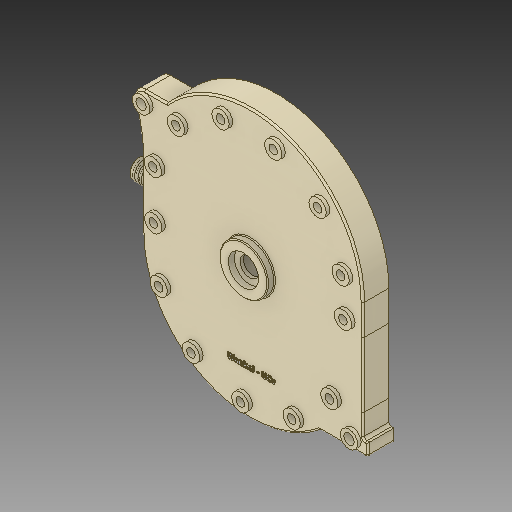
# Autodesk Inventor part: CapacFata
Saved by Autodesk Inventor 2019.4 (Build 234330000, 330)
## iProperties
Created: 2020-05-01
Part Number: CapacFata
Material: Aluminum 6061-AHC
Document SubType Name: Modeling
Designer: Gabriel
Density: 2.7 g/cm^3
Appearance: Light Beige
Author: Gabriel
Autodesk Inventor part; units mm, degrees
sketch "Sketch1" plane through (0, 0, 0) normal (0, 0, 1) x (1, 0, 0)
  arc A0 (-129.637, -28.0388) -> (75.3644, -124.0845) centre (-4.637, -28.0388) ccw projected
  line L0 (128.3644, -124.0845) -> (75.3644, -124.0845) projected
  line L1 (-129.637, -28.0388) -> (-129.637, 41.9612) projected
  arc A1 (-129.637, 41.9612) -> (-138.5073, 99.3374) centre (-319.637, 41.9612) ccw projected
  arc A2 (-127.0676, 114.9612) -> (-138.5073, 99.3374) centre (-127.0676, 102.9612) ccw projected
  line L2 (-127.0676, 114.9612) -> (-101.2341, 114.9612) projected
  arc A3 (125.363, 27.9662) -> (-101.2341, 114.9612) centre (-4.637, 27.9612) ccw projected
  line L3 (125.363, 27.9662) -> (125.3643, -7.0846) projected
  line L4 (125.3644, -106.0845) -> (125.3644, -82.0845) projected
  arc A4 (125.3644, -106.0845) -> (128.3644, -109.0845) centre (128.3644, -106.0845) ccw projected
  line L5 (131.3644, -109.0845) -> (131.3644, -121.0845) projected
  line L6 (131.3644, -109.0845) -> (128.3644, -109.0845) projected
  arc A5 (128.3644, -124.0845) -> (131.3644, -121.0845) centre (128.3644, -121.0845) ccw projected
  circle A6 centre (113.3644, -112.0845) radius 6 projected
  circle A7 centre (-127.0676, 102.9612) radius 6 projected
  line L7 (125.3643, -7.0846) -> (125.3644, -82.0845)
  constraints: 2 end point
extrude "Extrusion1" add sketch "Sketch1" along normal blind 30
ref_plane "Work Plane1" through (0, 0, 14) normal (0, 0, 1) x (1, 0, 0)
sketch "Sketch2" plane through (0, 0, 14) normal (0, 0, 1) x (1, 0, 0)
  circle A0 centre (-86.7234, 101.7852) radius 5 projected
  circle A1 centre (-35.1294, 134.0667) radius 5 projected
  circle A2 centre (25.7313, 134.1022) radius 5 projected
  circle A3 centre (77.1089, 101.5656) radius 5 projected
  circle A4 centre (103.6918, 47.0625) radius 5 projected
  circle A5 centre (106.363, 3.9612) radius 5 projected
  circle A6 centre (90.6258, -83.0388) radius 5 projected
  circle A7 centre (47.0048, -125.1631) radius 5 projected
  circle A8 centre (-12.3102, -137.7709) radius 5 projected
  circle A9 centre (-69.2934, -117.0307) radius 5 projected
  circle A10 centre (-106.6272, -69.2455) radius 5 projected
  circle A11 centre (-112.9659, -8.9375) radius 5 projected
  circle A12 centre (-113.371, 47.0684) radius 5 projected
extrude "Extrusion2" cut sketch "Sketch2" against normal through all
sketch "Sketch3" plane through (0, 0, 14) normal (0, 0, 1) x (1, 0, 0)
  circle A0 centre (-86.7234, 101.7852) radius 5 projected
  circle A1 centre (25.7313, 134.1022) radius 5 projected
  circle A2 centre (77.1089, 101.5656) radius 5 projected
  circle A3 centre (-35.1294, 134.0667) radius 5 projected
  circle A4 centre (-113.371, 47.0684) radius 5 projected
  line L0 (96.363, 34.1163) -> (96.363, 14.2081) projected
  arc A5 (96.363, 14.2081) -> (99.5937, 12.6317) centre (98.363, 14.2081) ccw projected
  arc A6 (112.2861, 13.2303) -> (99.5937, 12.6317) centre (106.363, 3.9612) ccw projected
  arc A7 (112.2861, 13.2303) -> (115.363, 14.9156) centre (113.363, 14.9156) ccw projected
  line L1 (115.363, 14.9156) -> (115.363, 36.9398) projected
  arc A8 (115.363, 36.9398) -> (111.9814, 38.3859) centre (113.363, 36.9398) ccw projected
  arc A9 (99.1242, 35.9658) -> (111.9814, 38.3859) centre (103.6918, 47.0625) ccw projected
  arc A10 (99.1242, 35.9658) -> (96.363, 34.1163) centre (98.363, 34.1163) ccw projected
  line L2 (118.363, -28.0388) -> (118.363, 27.9612) projected
  arc A11 (-127.637, -28.0388) -> (118.363, -28.0388) centre (-4.637, -28.0388) ccw projected
  line L3 (-127.637, 27.9612) -> (-127.637, -28.0388) projected
  arc A12 (118.363, 27.9612) -> (-127.637, 27.9612) centre (-4.637, 27.9612) ccw projected
  line L4 (115.363, -10.6889) -> (115.363, -8.6879) projected
  arc A13 (115.363, -8.6879) -> (111.0773, -5.9774) centre (112.363, -8.6879) ccw projected
  arc A14 (100.863, -5.5651) -> (111.0773, -5.9774) centre (106.363, 3.9612) ccw projected
  arc A15 (100.863, -5.5651) -> (96.363, -8.1632) centre (99.363, -8.1632) ccw projected
  line L5 (96.363, -8.1632) -> (96.363, -28.0388) projected
  arc A16 (88.1817, -67.8595) -> (96.363, -28.0388) centre (-4.637, -28.0388) ccw projected
  arc A17 (88.1817, -67.8595) -> (90.8716, -72.0416) centre (90.9387, -69.0423) ccw projected
  arc A18 (99.8396, -77.03) -> (90.8716, -72.0416) centre (90.6258, -83.0388) ccw projected
  arc A19 (99.8396, -77.03) -> (105.0958, -76.6054) centre (102.3524, -75.3913) ccw projected
  arc A20 (105.0958, -76.6054) -> (115.363, -28.0388) centre (-4.637, -28.0388) ccw projected
  line L6 (115.363, -28.0388) -> (115.363, -22.0845) projected
  line L7 (109.363, -22.0845) -> (115.363, -22.0845) projected
  line L8 (109.363, -12.6889) -> (109.363, -22.0845) projected
  arc A21 (111.363, -10.6889) -> (109.363, -12.6889) centre (111.363, -12.6889) ccw projected
  line L9 (115.363, -10.6889) -> (111.363, -10.6889) projected
  line L10 (-105.637, 4.3764) -> (-105.637, 33.9465) projected
  arc A22 (-105.637, 33.9465) -> (-109.6029, 36.7868) centre (-108.637, 33.9465) ccw projected
  arc A23 (-119.8172, 38.4561) -> (-109.6029, 36.7868) centre (-113.1445, 47.2011) ccw projected
  arc A24 (-119.8172, 38.4561) -> (-124.637, 36.0711) centre (-121.637, 36.0711) ccw projected
  line L11 (-124.637, 36.0711) -> (-124.637, 2.0539) projected
  arc A25 (-124.637, 2.0539) -> (-119.7789, -0.3014) centre (-121.637, 2.0539) ccw projected
  arc A26 (-109.5646, 1.5234) -> (-119.7789, -0.3014) centre (-112.9659, -8.9375) ccw projected
  arc A27 (-109.5646, 1.5234) -> (-105.637, 4.3764) centre (-108.637, 4.3764) ccw projected
  arc A28 (-119.5689, -17.7352) -> (-108.6305, -19.0472) centre (-112.9659, -8.9375) ccw projected
  arc A29 (-119.5689, -17.7352) -> (-124.3629, -19.932) centre (-121.3697, -20.1346) ccw projected
  arc A30 (-124.3629, -19.932) -> (-120.0611, -60.8609) centre (-4.637, -28.0388) ccw projected
  arc A31 (-120.0611, -60.8609) -> (-114.9151, -62.0129) centre (-117.1755, -60.0404) ccw projected
  arc A32 (-104.4886, -58.4555) -> (-114.9151, -62.0129) centre (-106.6272, -69.2455) ccw projected
  arc A33 (-104.4886, -58.4555) -> (-101.014, -54.7125) centre (-103.9053, -55.5127) ccw projected
  arc A34 (-104.4537, -21.9859) -> (-101.014, -54.7125) centre (-4.637, -28.0388) ccw projected
  arc A35 (-104.4537, -21.9859) -> (-108.6305, -19.0472) centre (-107.4482, -21.8043) ccw projected
  arc A36 (-107.5648, -80.2055) -> (-97.5934, -75.5216) centre (-106.6272, -69.2455) ccw projected
  arc A37 (-107.5648, -80.2055) -> (-110.4663, -84.6088) centre (-107.8206, -83.1946) ccw projected
  arc A38 (-110.4663, -84.6088) -> (-85.1291, -117.039) centre (-4.637, -28.0388) ccw projected
  arc A39 (-85.1291, -117.039) -> (-80.1546, -115.289) centre (-83.1168, -114.814) ccw projected
  arc A40 (-73.1976, -106.7468) -> (-80.1546, -115.289) centre (-69.2934, -117.0307) ccw projected
  arc A41 (-73.1976, -106.7468) -> (-72.2344, -101.7314) centre (-74.2623, -103.9422) ccw projected
  arc A42 (-92.4939, -75.8004) -> (-72.2344, -101.7314) centre (-4.637, -28.0388) ccw projected
  arc A43 (-92.4939, -75.8004) -> (-97.5934, -75.5216) centre (-95.1296, -77.2333) ccw projected
  arc A44 (-64.2806, -126.8221) -> (-58.3064, -117.5659) centre (-69.2934, -117.0307) ccw projected
  arc A45 (-64.2806, -126.8221) -> (-64.4078, -132.0939) centre (-62.9135, -129.4925) ccw projected
  arc A46 (-64.4078, -132.0939) -> (-25.7353, -146.1695) centre (-4.637, -28.0388) ccw projected
  arc A47 (-25.7353, -146.1695) -> (-22.4441, -142.0494) centre (-25.2078, -143.2163) ccw projected
  arc A48 (-21.0708, -131.1186) -> (-22.4441, -142.0494) centre (-12.3102, -137.7709) ccw projected
  arc A49 (-21.0708, -131.1186) -> (-22.9118, -126.3548) centre (-23.46, -129.3043) ccw projected
  arc A50 (-53.8341, -115.1) -> (-22.9118, -126.3548) centre (-4.637, -28.0388) ccw projected
  arc A51 (-53.8341, -115.1) -> (-58.3064, -117.5659) centre (-55.31, -117.7118) ccw projected
  arc A52 (-2.8705, -143.4181) -> (-2.7091, -132.4025) centre (-12.3102, -137.7709) ccw projected
  arc A53 (-2.8705, -143.4181) -> (-0.1847, -147.9562) centre (-0.296, -144.9583) ccw projected
  arc A54 (-0.1847, -147.9562) -> (40.0704, -139.3997) centre (-4.637, -28.0388) ccw projected
  arc A55 (40.0704, -139.3997) -> (40.6782, -134.1615) centre (38.9527, -136.6157) ccw projected
  arc A56 (36.0503, -124.1639) -> (40.6782, -134.1615) centre (47.0048, -125.1631) ccw projected
  arc A57 (36.0503, -124.1639) -> (31.9647, -121.0996) centre (33.0627, -123.8915) ccw projected
  arc A58 (-0.2231, -127.9414) -> (31.9647, -121.0996) centre (-4.637, -28.0388) ccw projected
  arc A59 (-0.2231, -127.9414) -> (-2.7091, -132.4025) centre (-0.0907, -130.9384) ccw projected
  arc A60 (80.8064, -87.9965) -> (90.0289, -94.0226) centre (90.6258, -83.0388) ccw projected
  arc A61 (80.8064, -87.9965) -> (75.7177, -87.5629) centre (78.1283, -89.3487) ccw projected
  arc A62 (52.0465, -110.4219) -> (75.7177, -87.5629) centre (-4.637, -28.0388) ccw projected
  arc A63 (52.0465, -110.4219) -> (52.3022, -115.5226) centre (53.747, -112.8934) ccw projected
  arc A64 (58.0028, -124.9499) -> (52.3022, -115.5226) centre (47.0048, -125.1631) ccw projected
  arc A65 (58.0028, -124.9499) -> (62.6853, -127.3752) centre (61.0022, -124.8917) ccw projected
  arc A66 (62.6853, -127.3752) -> (92.2893, -98.7869) centre (-4.637, -28.0388) ccw projected
  arc A67 (92.2893, -98.7869) -> (90.0289, -94.0226) centre (89.8661, -97.0182) ccw projected
  arc A68 (-105.5908, 54.8446) -> (-116.2183, 57.6935) centre (-113.371, 47.0684) ccw projected
  arc A69 (-105.5908, 54.8446) -> (-100.5904, 56.1206) centre (-103.469, 56.9654) ccw projected
  arc A70 (-86.0788, 85.9891) -> (-100.5904, 56.1206) centre (-4.637, 27.9612) ccw projected
  arc A71 (-86.0788, 85.9891) -> (-88.0637, 90.6947) centre (-88.522, 87.7299) ccw projected
  arc A72 (-96.6447, 97.6037) -> (-88.0637, 90.6947) centre (-86.383, 101.5656) ccw projected
  arc A73 (-96.6447, 97.6037) -> (-101.8743, 98.2812) centre (-99.4434, 96.5232) ccw projected
  arc A74 (-101.8743, 98.2812) -> (-119.8758, 61.4279) centre (-4.637, 27.9612) ccw projected
  arc A75 (-119.8758, 61.4279) -> (-116.2183, 57.6935) centre (-116.9948, 60.5913) ccw projected
  arc A76 (-76.0047, 104.257) -> (-83.5076, 112.3047) centre (-86.7234, 101.7852) ccw projected
  arc A77 (-76.0047, 104.257) -> (-71.0879, 102.6893) centre (-73.0814, 104.9311) ccw projected
  arc A78 (-42.9535, 120.3292) -> (-71.0879, 102.6893) centre (-4.637, 27.9612) ccw projected
  arc A79 (-42.9535, 120.3292) -> (-42.1431, 125.3716) centre (-44.1029, 123.1002) ccw projected
  arc A80 (-45.7591, 135.7781) -> (-42.1431, 125.3716) centre (-34.9571, 133.7) ccw projected
  arc A81 (-45.7591, 135.7781) -> (-49.835, 139.1239) centre (-48.705, 136.3448) ccw projected
  arc A82 (-49.835, 139.1239) -> (-84.6304, 117.4098) centre (-4.637, 27.9612) ccw projected
  arc A83 (-84.6304, 117.4098) -> (-83.5076, 112.3047) centre (-82.6306, 115.1736) ccw projected
  arc A84 (-24.7296, 130.4828) -> (-26.8278, 141.2836) centre (-35.1294, 134.0667) ccw projected
  arc A85 (-24.7296, 130.4828) -> (-21.3907, 126.5478) centre (-21.8933, 129.5054) ccw projected
  arc A86 (11.8164, 126.5983) -> (-21.3907, 126.5478) centre (-4.637, 27.9612) ccw projected
  arc A87 (11.8164, 126.5983) -> (15.1757, 130.4451) centre (12.31, 129.5574) ccw projected
  arc A88 (17.6238, 141.1864) -> (15.1757, 130.4451) centre (25.6831, 133.7) ccw projected
  arc A89 (17.6238, 141.1864) -> (15.9402, 146.1838) centre (15.4258, 143.2282) ccw projected
  arc A90 (15.9402, 146.1838) -> (-25.0747, 146.208) centre (-4.637, 27.9612) ccw projected
  arc A91 (-25.0747, 146.208) -> (-26.8278, 141.2836) centre (-24.5637, 143.2518) ccw projected
  arc A92 (32.6517, 125.5519) -> (36.5958, 135.8233) centre (25.7313, 134.1022) ccw projected
  arc A93 (32.6517, 125.5519) -> (33.398, 120.4454) centre (34.539, 123.22) ccw projected
  arc A94 (61.586, 102.8912) -> (33.398, 120.4454) centre (-4.637, 27.9612) ccw projected
  arc A95 (61.586, 102.8912) -> (66.4733, 104.3734) centre (63.5727, 105.1391) ccw projected
  arc A96 (74.2414, 112.1852) -> (66.4733, 104.3734) centre (77.1089, 101.5656) ccw projected
  arc A97 (74.2414, 112.1852) -> (75.4619, 117.3154) centre (73.4594, 115.0815) ccw projected
  arc A98 (75.4619, 117.3154) -> (40.6921, 139.0705) centre (-4.637, 27.9612) ccw projected
  arc A99 (40.6921, 139.0705) -> (36.5958, 135.8233) centre (39.5589, 136.2927) ccw projected
  arc A100 (106.8876, 57.588) -> (96.1602, 55.0797) centre (103.6918, 47.0625) ccw projected
  arc A101 (106.8876, 57.588) -> (110.6412, 61.2919) centre (107.7592, 60.4586) ccw projected
  arc A102 (110.6412, 61.2919) -> (92.6832, 98.1664) centre (-4.637, 27.9612) ccw projected
  arc A103 (92.6832, 98.1664) -> (87.4887, 97.5834) centre (90.2502, 96.4113) ccw projected
  arc A104 (78.7008, 90.9628) -> (87.4887, 97.5834) centre (77.363, 101.8811) ccw projected
  arc A105 (78.7008, 90.9628) -> (76.6277, 86.2368) centre (79.0656, 87.9851) ccw projected
  arc A106 (91.2302, 56.4126) -> (76.6277, 86.2368) centre (-4.637, 27.9612) ccw projected
  arc A107 (91.2302, 56.4126) -> (96.1602, 55.0797) centre (94.1062, 57.2662) ccw projected
  circle A108 centre (106.363, 3.9612) radius 5 projected
  circle A109 centre (-112.9659, -8.9375) radius 5 projected
  circle A110 centre (-106.6272, -69.2455) radius 5 projected
  circle A111 centre (-69.2934, -117.0307) radius 5 projected
  circle A112 centre (-12.3102, -137.7709) radius 5 projected
  circle A113 centre (47.0048, -125.1631) radius 5 projected
  circle A114 centre (90.6258, -83.0388) radius 5 projected
  circle A115 centre (103.6918, 47.0625) radius 5 projected
  line L12 (-102.637, 27.9612) -> (-102.637, -28.0388) projected
  arc A116 (-102.637, -28.0388) -> (93.363, -28.0388) centre (-4.637, -28.0388) ccw projected
  line L13 (93.363, -28.0388) -> (93.363, 27.9612) projected
  arc A117 (93.363, 27.9612) -> (-102.637, 27.9612) centre (-4.637, 27.9612) ccw projected
extrude "Extrusion3" cut sketch "Sketch3" against normal blind 30 contours A10 A9 A8 L1 A7 A6 A5 L0 | L9 A21 L8 L7 L6 A20 A19 A18 A17 A16 L5 A15 A14 A13 L4 | A27 A26 A25 L11 A24 A23 A22 L10 | A28 A35 A34 A33 A32 A31 A30 A29 | A36 A43 A42 A41 A40 A39 A38 A37 | A44 A51 A50 A49 A48 A47 A46 A45 | A52 A59 A58 A57 A56 A55 A54 A53 | A60 A67 A66 A65 A64 A63 A62 A61 | A68 A75 A74 A73 A72 A71 A70 A69 | A76 A83 A82 A81 A80 A79 A78 A77 | A84 A91 A90 A89 A88 A87 A86 A85 | A92 A99 A98 A97 A96 A95 A94 A93 | A100 A107 A106 A105 A104 A103 A102 A101
sketch "Sketch4" plane through (0, 0, 30) normal (0, 0, 1) x (1, 0, 0)
  circle A0 centre (-4.637, -0.0388) radius 19.5 construction
  circle A1 centre (-4.637, -0.0388) radius 11
  dimension "d7" = 22
  constraints: 1 centre point, 1 coincident
  measures "d7" diameter of A1
extrude "Extrusion4" cut sketch "Sketch4" against normal through all
sketch "Sketch5" plane through (0, 0, 14) normal (0, 0, 1) x (1, 0, 0)
  arc A0 (125.363, 27.9662) -> (-101.2341, 114.9612) centre (-4.637, 27.9612) ccw construction
  arc A1 (-129.637, -28.0388) -> (75.3644, -124.0845) centre (-4.637, -28.0388) ccw construction
  line L0 (-129.637, -28.0388) -> (-129.637, 41.9612) construction
  line L1 (125.363, 27.9662) -> (125.3643, -7.0846) construction
  arc A2 (75.3644, -124.0845) -> (125.3643, -7.0846) centre (-36.5111, -7.0908) ccw construction
  arc A3 (-101.2341, 114.9612) -> (-129.637, 41.9612) centre (-21.6247, 41.9612) ccw construction
  arc A4 (115.363, 27.9658) -> (-124.637, 27.9612) centre (-4.637, 27.9612) ccw
  line L2 (115.363, 27.9658) -> (115.3651, -27.8528)
  arc A5 (-124.637, -28.7808) -> (115.3651, -27.8528) centre (-4.637, -28.0388) ccw
  line L3 (-124.637, -28.7808) -> (-124.637, 27.9612)
  line L4 (-104.637, 27.9612) -> (-104.637, -28.7161)
  arc A6 (-104.637, -28.7161) -> (95.3651, -27.8694) centre (-4.637, -28.0388) ccw
  line L5 (95.3651, -27.8694) -> (95.363, 27.965)
  arc A7 (95.363, 27.965) -> (-104.637, 27.9612) centre (-4.637, 27.9612) ccw
  dimension "d10" = 10
  dimension "d139" = 5
  dimension "d140" = 120.0023
  dimension "d141" = 20
  constraints: 12 point on circle, 8 end point, 6 centre point, 2 tangent, 1 concentric, 1 parallel, 4 other
  measures "d10" radial gap between concentric circles of A4 A0
  measures "d139" distance between parallel lines of L3 L0
  measures "d140" radius of A5
  measures "d141" distance between parallel lines of L2 L5
extrude "Extrusion8" cut sketch "Sketch5" along normal blind 10
hole "Hole1" at (103.6918, 47.0625, 0) direction (0, 0, 1) diameter 10 end through all
hole "Hole2" at (77.1089, 101.5656, 0) direction (0, 0, 1) diameter 10 end through all
hole "Hole3" at (25.7313, 134.1022, 0) direction (0, 0, 1) diameter 10 end through all
hole "Hole4" at (-35.1294, 134.0667, 0) direction (0, 0, 1) diameter 10 end through all
hole "Hole5" at (-86.7234, 101.7852, 0) direction (0, 0, 1) diameter 10 end through all
hole "Hole6" at (-113.371, 47.0684, 0) direction (0, 0, 1) diameter 10 end through all
hole "Hole7" at (-112.9659, -8.9375, 0) direction (0, 0, 1) diameter 10 end through all
hole "Hole8" at (-106.6272, -69.2455, 0) direction (0, 0, 1) diameter 10 end through all
hole "Hole9" at (-69.2934, -117.0307, 0) direction (0, 0, 1) diameter 10 end through all
hole "Hole10" at (-12.3102, -137.7709, 0) direction (0, 0, 1) diameter 10 end through all
hole "Hole11" at (47.0048, -125.1631, 0) direction (0, 0, 1) diameter 10 end through all
hole "Hole12" at (90.6258, -83.0388, 0) direction (0, 0, 1) diameter 10 end through all
hole "Hole13" at (106.363, 3.9612, 0) direction (0, 0, 1) diameter 10 end through all
sketch "Sketch6" plane through (0, 0, 0) normal (0, 0, -1) x (-1, 0, 0)
  circle A0 centre (-25.7313, 134.1022) radius 5 projected
  circle A1 centre (35.1294, 134.0667) radius 5 projected
  circle A2 centre (86.7234, 101.7852) radius 5 projected
  circle A3 centre (113.371, 47.0684) radius 5 projected
  circle A4 centre (112.9659, -8.9375) radius 5 projected
  circle A5 centre (106.6272, -69.2455) radius 5 projected
  circle A6 centre (69.2934, -117.0307) radius 5 projected
  circle A7 centre (12.3102, -137.7709) radius 5 projected
  circle A8 centre (-47.0048, -125.1631) radius 5 projected
  circle A9 centre (-90.6258, -83.0388) radius 5 projected
  circle A10 centre (-106.363, 3.9612) radius 5 projected
  circle A11 centre (-103.6918, 47.0625) radius 5 projected
  circle A12 centre (-77.1089, 101.5656) radius 5 projected
  circle A13 centre (-25.7313, 134.1022) radius 8
  circle A14 centre (35.1294, 134.0667) radius 8
  circle A15 centre (86.7234, 101.7852) radius 8
  circle A16 centre (113.371, 47.0684) radius 8
  circle A17 centre (112.9659, -8.9375) radius 8
  circle A18 centre (106.6272, -69.2455) radius 8
  circle A19 centre (69.2934, -117.0307) radius 8
  circle A20 centre (12.3102, -137.7709) radius 8
  circle A21 centre (-47.0048, -125.1631) radius 8
  circle A22 centre (-90.6258, -83.0388) radius 8
  circle A23 centre (-106.363, 3.9612) radius 8
  circle A24 centre (-103.6918, 47.0625) radius 8
  circle A25 centre (-77.1089, 101.5656) radius 8
  dimension "d14" = 16
  constraints: 13 centre point, 13 coincident, 12 equal radius
  measures "d14" diameter of A13
extrude "Extrusion6" add sketch "Sketch6" against normal up to surface (30 mm away)
sketch "Sketch7" plane through (0, 0, 0) normal (0, 0, -1) x (-1, 0, 0)
  line L0 (-106.8821, -23.6279) -> (-115.363, -23.6279)
  line L1 (-115.363, -23.6279) -> (-115.363, -9.7728)
  line L2 (-115.363, -9.7728) -> (-106.8821, -9.7728)
  line L3 (-106.8821, -9.7728) -> (-106.8821, -23.6279)
  line L4 (-115.363, -28.0388) -> (-115.363, -22.0845) projected
  constraints: 8 end point, 2 parallel, 1 collinear, 1 horizontal, 1 perpendicular
extrude "Extrusion7" cut sketch "Sketch7" against normal blind 20
sketch "Sketch8" plane through (0, 0, 0) normal (0, 0, -1) x (-1, 0, 0)
  circle A0 centre (4.637, -0.0388) radius 31.5
  circle A1 centre (4.637, -0.0388) radius 11 projected
  dimension "d144" = 63
  constraints: 1 centre point, 1 concentric
  measures "d144" diameter of A0
extrude "Extrusion9" cut sketch "Sketch8" against normal blind 1
sketch "Sketch9" plane through (-4.637, -0.0388, 1) normal (0, 0, -1) x (-1, 0, 0)
  circle A0 centre (0, 0) radius 27
  dimension "d147" = 54
  constraints: 1 centre point
  measures "d147" diameter of A0
extrude "Extrusion10" cut sketch "Sketch9" against normal blind 6
sketch "Sketch10" plane through (-4.637, -0.0388, 7) normal (0, 0, -1) x (-1, 0, 0)
  circle A0 centre (0, 0) radius 24 construction
  circle A1 centre (0, 0) radius 27 projected
  point P0 (0, 24)
  dimension "d150" = 48
  constraints: 2 vertical alignment, 3 other
hole "Hole14" at (-4.637, 23.9612, 7) direction (0, 0, 1) diameter 3.242 depth 9 tip angle 118 thread size "M4x0.7" class "6H" standard "ISO Metric profile"
pattern_circular "Circular Pattern1" count 6 over 360 about axis through (-4.637, -0.0388, 30) along (0, 0, -1) of "Hole14"
sketch "Sketch11" plane through (0, 0, 30) normal (0, 0, 1) x (1, 0, 0)
  circle A0 centre (-4.637, -0.0388) radius 28
  circle A1 centre (-4.637, -0.0388) radius 11 projected
  dimension "d161" = 56
  constraints: 1 centre point, 1 concentric
  measures "d161" diameter of A0
extrude "Extrusion11" add sketch "Sketch11" along normal blind 8
sketch "Sketch12" plane through (-4.637, -0.0388, 38) normal (0, 0, 1) x (1, 0, 0)
  circle A0 centre (0, 0) radius 17.5
  circle A1 centre (0, 0) radius 11 projected
  dimension "d164" = 35
  constraints: 1 centre point, 1 concentric
  measures "d164" diameter of A0
extrude "Extrusion12" cut sketch "Sketch12" against normal blind 7
sketch "Sketch13" plane through (-4.637, -0.0388, 7) normal (0, 0, -1) x (-1, 0, 0)
  circle A0 centre (0, 0) radius 19.5
  circle A1 centre (0, 0) radius 11 projected
  dimension "d167" = 39
  constraints: 1 centre point, 1 concentric
  measures "d167" diameter of A0
extrude "Extrusion13" cut sketch "Sketch13" against normal blind 20
fillet "Fillet1" radius 2 14 edges at (125.3636, 10.4408, 30) (125.3644, -44.5845, 30) (125.3644, -94.0845, 30) (126.2431, -108.2058, 30) (129.8644, -109.0845, 30) (41.9567, 149.3244, 30) (-136.7496, 110.0504, 30) (-131.8677, 70.9901, 30) (-129.637, 6.9612, 30) (-57.6692, -141.2315, 30) (-114.1508, 114.9612, 30) (130.4857, -123.2058, 30) (131.3644, -115.0845, 30) (101.8644, -124.0845, 30)
chamfer "Chamfer1" distance 1 angle 45 1 edges at (-32.637, -0.0388, 38)
fillet "Fillet2" radius 1 1 edges at (-32.637, -0.0388, 30)
sketch "Sketch14" plane through (0, 0, 30) normal (0, 0, 1) x (1, 0, 0)
  circle A0 centre (-86.7234, 101.7852) radius 10
  circle A1 centre (-86.7234, 101.7852) radius 5 projected
  circle A2 centre (-35.1294, 134.0667) radius 5 projected
  circle A3 centre (25.7313, 134.1022) radius 5 projected
  circle A4 centre (77.1089, 101.5656) radius 5 projected
  circle A5 centre (103.6918, 47.0625) radius 5 projected
  circle A6 centre (106.363, 3.9612) radius 5 projected
  circle A7 centre (90.6258, -83.0388) radius 5 projected
  circle A8 centre (47.0048, -125.1631) radius 5 projected
  circle A9 centre (113.3644, -112.0845) radius 6 projected
  circle A10 centre (-12.3102, -137.7709) radius 5 projected
  circle A11 centre (-69.2934, -117.0307) radius 5 projected
  circle A12 centre (-106.6272, -69.2455) radius 5 projected
  circle A13 centre (-112.9659, -8.9375) radius 5 projected
  circle A14 centre (-113.371, 47.0684) radius 5 projected
  circle A15 centre (-127.0676, 102.9612) radius 6 projected
  circle A16 centre (-35.1294, 134.0667) radius 10
  circle A17 centre (25.7313, 134.1022) radius 10
  circle A18 centre (77.1089, 101.5656) radius 10
  circle A19 centre (103.6918, 47.0625) radius 10
  circle A20 centre (106.363, 3.9612) radius 10
  circle A21 centre (90.6258, -83.0388) radius 10
  circle A22 centre (113.3644, -112.0845) radius 10
  circle A23 centre (47.0048, -125.1631) radius 10
  circle A24 centre (-12.3102, -137.7709) radius 10
  circle A25 centre (-69.2934, -117.0307) radius 10
  circle A26 centre (-106.6272, -69.2455) radius 10
  circle A27 centre (-112.9659, -8.9375) radius 10
  circle A28 centre (-113.371, 47.0684) radius 10
  circle A29 centre (-127.0676, 102.9612) radius 10
  dimension "d175" = 20
  constraints: 15 centre point, 14 coincident, 14 equal radius, 1 concentric
  measures "d175" diameter of A0
extrude "Extrusion14" add sketch "Sketch14" along normal blind 4
sketch "Sketch15" plane through (-129.637, -28.0388, 0) normal (-1, 0, 0) x (0, 0, 1)
  circle A0 centre (14, 46.2022) radius 11
  line L0 (0, 0) -> (0, 70) projected
  dimension "d178" = 22
  dimension "d179" = 14
  constraints: 1 centre point
  measures "d178" diameter of A0
  measures "d179" distance from line of L0 A0.centre
extrude "Extrusion15" add sketch "Sketch15" along normal blind 20
sketch "Sketch16" plane through (-149.637, 18.1634, 14) normal (-1, 0, 0) x (0, 0, 1)
  circle A0 centre (0, 0) radius 7.5
  circle A1 centre (0, 0) radius 11 projected
  dimension "d182" = 15
  constraints: 1 centre point, 1 concentric
  measures "d182" diameter of A0
extrude "Extrusion16" cut sketch "Sketch16" against normal blind 30 contours A0
chamfer "Chamfer2" distance 1 angle 45 1 edges at (-149.637, 18.1634, 3)
fillet "Fillet3" radius 1 1 edges at (-129.637, 18.1634, 3)
ref_plane "Work Plane2" through (-149.637, 18.1634, 14) normal (0, 1, 0) x (1, 0, 0)
sketch "Sketch17" plane through (-149.637, 18.1634, 14) normal (0, 1, 0) x (1, 0, 0)
  arc A0 (12, -11) -> (14, -11) centre (13, -11) ccw
  arc A1 (8, -11) -> (10, -11) centre (9, -11) ccw
  arc A2 (4, -11) -> (6, -11) centre (5, -11) ccw
  line L0 (15, -8) -> (3, -8)
  line L1 (3, -8) -> (3, -11)
  line L2 (15, -11) -> (15, -8)
  line L3 (3, -11) -> (4, -11)
  line L4 (6, -11) -> (8, -11)
  line L5 (10, -11) -> (12, -11)
  line L6 (14, -11) -> (15, -11)
  line L7 (-56.2003, 0) -> (337.2017, 0) projected
  line L8 (0, -7.5) -> (0, 7.5) projected
  dimension "d190" = 2
  dimension "d191" = 4
  dimension "d192" = 4
  dimension "d193" = 3
  dimension "d194" = 12
  dimension "d195" = 1
  dimension "d196" = 8
  dimension "d197" = 2
  dimension "d198" = 3
  constraints: 14 end point, 6 point on circle, 5 parallel, 3 centre point, 3 collinear, 2 equal radius, 2 horizontal alignment, 1 horizontal, 1 perpendicular
  measures "d190" diameter of A0
  measures "d191" distance of A0.centre A1.centre
  measures "d192" distance of A2.centre A1.centre
  measures "d193" distance of L0.end L1.end
  measures "d194" distance of L0.start L0.end
  measures "d195" distance of L1.end L3.end
  measures "d196" distance between parallel lines of L0 L7
  measures "d197" distance from line of L2 A0.centre
  measures "d198" distance between parallel lines of L8 L1
revolve "Revolution1" add sketch "Sketch17" angle 360 about axis through (-149.637, 18.1634, 14) along (1, 0, 0)
sketch "Sketch18" plane through (0, 0, 0) normal (0, 0, -1) x (-1, 0, 0)
  arc A0 (-40.6782, -134.1615) -> (-36.0503, -124.1639) centre (-47.0048, -125.1631) ccw projected
  arc A1 (-31.9647, -121.0996) -> (-36.0503, -124.1639) centre (-33.0627, -123.8915) ccw projected
  arc A2 (-40.6782, -134.1615) -> (-40.0704, -139.3997) centre (-38.9527, -136.6157) ccw projected
  arc A3 (58.3064, -117.5659) -> (53.8341, -115.1) centre (55.31, -117.7118) ccw projected
  arc A4 (58.3064, -117.5659) -> (64.2806, -126.8221) centre (69.2934, -117.0307) ccw projected
  arc A5 (64.4078, -132.0939) -> (64.2806, -126.8221) centre (62.9135, -129.4925) ccw projected
  line L0 (-31.9647, -121.0996) -> (-33.2623, -116.03)
  line L1 (-33.2623, -116.03) -> (-45.9654, -139.3997)
  line L2 (-45.9654, -139.3997) -> (-40.0704, -139.3997)
  line L3 (53.8341, -115.1) -> (55.31, -110.1197)
  line L4 (55.31, -110.1197) -> (70.6918, -132.0939)
  line L5 (70.6918, -132.0939) -> (64.4078, -132.0939)
  constraints: 12 end point, 2 horizontal
extrude "Extrusion17" add sketch "Sketch18" against normal up to surface (24 mm away)
ref_plane "Work Plane3" through (-4.637, -0.0388, 7) normal (0.9848078, 0.1736482, 0) x (0, 0, 1)
sketch "Sketch19" plane through (-4.637, -0.0388, 7) normal (0.9848078, 0.1736482, 0) x (0, 0, 1)
  line L0 (7.6077, 17.4759) -> (10.6077, 17.4759)
  line L1 (10.6077, 17.4759) -> (10.6077, 157.4759)
  line L2 (10.6077, 157.4759) -> (7.6077, 157.4759)
  line L3 (7.6077, 157.4759) -> (7.6077, 17.4759)
  dimension "d203" = 140
  dimension "d204" = 3
  constraints: 8 end point, 2 parallel, 1 horizontal, 1 perpendicular
  measures "d203" distance of L2.end L0.start
  measures "d204" distance of L0.start L0.end
revolve "Revolution2" cut sketch "Sketch19" angle 360 about axis through (22.7084, -155.1223, 14.6077) along (-0.1736482, 0.9848078, 0)
thread "Thread1" size "M6x1" class "6H" standard "ANSI Metric M Profile" full length
sketch "Sketch20" plane through (0, 0, 30) normal (0, 0, 1) x (1, 0, 0)
  line L0 (-31.0066, -97.7863) -> (25.1461, -97.7863) construction
  line L1 (25.1461, -97.7863) -> (25.1461, -109.3185) construction
  line L2 (25.1461, -109.3185) -> (-31.0066, -109.3185) construction
  line L3 (-31.0066, -109.3185) -> (-31.0066, -97.7863) construction
  line L4 (-22.491, -98.0537) -> (-24.008, -104.0537)
  line L5 (-24.008, -104.0537) -> (-25.6612, -104.0537)
  line L6 (-25.6612, -104.0537) -> (-26.6239, -100.3438)
  line L7 (-26.6239, -100.3438) -> (-27.5526, -104.0537)
  line L8 (-27.5526, -104.0537) -> (-29.2106, -104.0537)
  line L9 (-29.2106, -104.0537) -> (-30.7277, -98.0537)
  line L10 (-30.7277, -98.0537) -> (-29.162, -98.0537)
  line L11 (-29.162, -98.0537) -> (-28.3354, -102.0699)
  line L12 (-28.3354, -102.0699) -> (-27.3338, -98.0537)
  line L13 (-27.3338, -98.0537) -> (-25.8362, -98.0537)
  line L14 (-25.8362, -98.0537) -> (-24.8832, -102.0748)
  line L15 (-24.8832, -102.0748) -> (-24.0178, -98.0537)
  line L16 (-24.0178, -98.0537) -> (-22.491, -98.0537)
  spline S0 degree 2 poles (-19.3354, -103.5723) (-19.4813, -103.6939) (-19.7098, -103.8884) (-19.9043, -103.9856) knots 0 0 0 1 2 2 2
  spline S1 degree 2 poles (-19.9043, -103.9856) (-20.0939, -104.078) (-20.4537, -104.1752) (-20.7747, -104.1752) knots 0 0 0 1 2 2 2
  spline S2 degree 2 poles (-20.7747, -104.1752) (-21.3776, -104.1752) (-22.1701, -103.3681) (-22.1701, -102.7555) knots 0 0 0 1 2 2 2
  spline S3 degree 2 poles (-22.1701, -102.7555) (-22.1701, -102.2547) (-21.7666, -101.6323) (-21.3873, -101.4524) knots 0 0 0 1 2 2 2
  spline S4 degree 2 poles (-21.3873, -101.4524) (-21.0032, -101.2676) (-19.9383, -101.1218) (-19.3257, -101.0829) knots 0 0 0 1 2 2 2
  line L17 (-19.3257, -101.0829) -> (-19.3257, -101.0585)
  spline S5 degree 2 poles (-19.3257, -101.0585) (-19.3257, -100.6842) (-19.88, -100.3973) (-20.4343, -100.3973) knots 0 0 0 1 2 2 2
  spline S6 degree 2 poles (-20.4343, -100.3973) (-20.6823, -100.3973) (-21.3533, -100.5772) (-21.6693, -100.7182) knots 0 0 0 1 2 2 2
  line L18 (-21.6693, -100.7182) -> (-21.7909, -100.7182)
  line L19 (-21.7909, -100.7182) -> (-21.7909, -99.6242)
  spline S7 degree 2 poles (-21.7909, -99.6242) (-21.5818, -99.5658) (-20.6482, -99.4005) (-20.1717, -99.4005) knots 0 0 0 1 2 2 2
  spline S8 degree 2 poles (-20.1717, -99.4005) (-19.0048, -99.4005) (-17.9351, -100.1785) (-17.9351, -100.9759) knots 0 0 0 1 2 2 2
  line L20 (-17.9351, -100.9759) -> (-17.9351, -104.0537)
  line L21 (-17.9351, -104.0537) -> (-19.3354, -104.0537)
  line L22 (-19.3354, -104.0537) -> (-19.3354, -103.5723)
  line L23 (-19.3354, -102.8722) -> (-19.3354, -101.9337)
  spline S9 degree 2 poles (-19.3354, -101.9337) (-19.6952, -101.9678) (-20.1377, -102.0213) (-20.3516, -102.0991) knots 0 0 0 1 2 2 2
  spline S10 degree 2 poles (-20.3516, -102.0991) (-20.5413, -102.1623) (-20.7455, -102.4248) (-20.7455, -102.6388) knots 0 0 0 1 2 2 2
  spline S11 degree 2 poles (-20.7455, -102.6388) (-20.7455, -102.9548) (-20.4003, -103.1931) (-20.0648, -103.1931) knots 0 0 0 1 2 2 2
  spline S12 degree 2 poles (-20.0648, -103.1931) (-19.88, -103.1931) (-19.491, -103.0229) (-19.3354, -102.8722) knots 0 0 0 1 2 2 2
  line L24 (-12.6547, -104.0537) -> (-14.0745, -104.0537)
  line L25 (-14.0745, -104.0537) -> (-14.0745, -101.8122)
  spline S13 degree 2 poles (-14.0745, -101.8122) (-14.0745, -101.535) (-14.1183, -100.9905) (-14.1766, -100.8641) knots 0 0 0 1 2 2 2
  spline S14 degree 2 poles (-14.1766, -100.8641) (-14.2495, -100.7085) (-14.5218, -100.5772) (-14.7552, -100.5772) knots 0 0 0 1 2 2 2
  spline S15 degree 2 poles (-14.7552, -100.5772) (-14.9254, -100.5772) (-15.2803, -100.7085) (-15.4797, -100.8495) knots 0 0 0 1 2 2 2
  line L26 (-15.4797, -100.8495) -> (-15.4797, -104.0537)
  line L27 (-15.4797, -104.0537) -> (-16.8897, -104.0537)
  line L28 (-16.8897, -104.0537) -> (-16.8897, -99.5269)
  line L29 (-16.8897, -99.5269) -> (-15.4797, -99.5269)
  line L30 (-15.4797, -99.5269) -> (-15.4797, -100.0278)
  spline S16 degree 2 poles (-15.4797, -100.0278) (-15.1345, -99.736) (-14.4781, -99.4054) (-14.0794, -99.4054) knots 0 0 0 1 2 2 2
  spline S17 degree 2 poles (-14.0794, -99.4054) (-13.3889, -99.4054) (-12.6547, -100.2806) (-12.6547, -101.1072) knots 0 0 0 1 2 2 2
  line L31 (-12.6547, -101.1072) -> (-12.6547, -104.0537)
  line L32 (-7.0777, -104.0537) -> (-8.7552, -104.0537)
  line L33 (-8.7552, -104.0537) -> (-9.9805, -102.0893)
  line L34 (-9.9805, -102.0893) -> (-10.1993, -102.3811)
  line L35 (-10.1993, -102.3811) -> (-10.1993, -104.0537)
  line L36 (-10.1993, -104.0537) -> (-11.6093, -104.0537)
  line L37 (-11.6093, -104.0537) -> (-11.6093, -97.7863)
  line L38 (-11.6093, -97.7863) -> (-10.1993, -97.7863)
  line L39 (-10.1993, -97.7863) -> (-10.1993, -101.2968)
  line L40 (-10.1993, -101.2968) -> (-8.8622, -99.5269)
  line L41 (-8.8622, -99.5269) -> (-7.1944, -99.5269)
  line L42 (-7.1944, -99.5269) -> (-8.7795, -101.4767)
  line L43 (-8.7795, -101.4767) -> (-7.0777, -104.0537)
  spline S18 degree 2 poles (-4.316, -104.1752) (-5.5996, -104.1752) (-6.9659, -102.95) (-6.9659, -101.8171) knots 0 0 0 1 2 2 2
  spline S19 degree 2 poles (-6.9659, -101.8171) (-6.9659, -100.7085) (-5.692, -99.3859) (-4.5445, -99.3859) knots 0 0 0 1 2 2 2
  spline S20 degree 2 poles (-4.5445, -99.3859) (-3.5089, -99.3859) (-2.4586, -100.5091) (-2.4586, -101.5496) knots 0 0 0 1 2 2 2
  line L44 (-2.4586, -101.5496) -> (-2.4586, -102.0602)
  line L45 (-2.4586, -102.0602) -> (-5.5559, -102.0602)
  spline S21 degree 2 poles (-5.5559, -102.0602) (-5.5364, -102.3762) (-5.3079, -102.7944) (-5.1231, -102.9208) knots 0 0 0 1 2 2 2
  spline S22 degree 2 poles (-5.1231, -102.9208) (-4.9432, -103.0472) (-4.457, -103.1542) (-4.1701, -103.1542) knots 0 0 0 1 2 2 2
  spline S23 degree 2 poles (-4.1701, -103.1542) (-3.927, -103.1542) (-3.4505, -103.0472) (-3.2512, -102.9548) knots 0 0 0 1 2 2 2
  spline S24 degree 2 poles (-3.2512, -102.9548) (-3.0761, -102.8819) (-2.7844, -102.702) (-2.692, -102.6339) knots 0 0 0 1 2 2 2
  line L46 (-2.692, -102.6339) -> (-2.5413, -102.6339)
  line L47 (-2.5413, -102.6339) -> (-2.5413, -103.8008)
  spline S25 degree 2 poles (-2.5413, -103.8008) (-2.7163, -103.8689) (-2.9983, -103.9856) (-3.2512, -104.044) knots 0 0 0 1 2 2 2
  spline S26 degree 2 poles (-3.2512, -104.044) (-3.4797, -104.1072) (-3.9659, -104.1752) (-4.316, -104.1752) knots 0 0 0 1 2 2 2
  spline S27 degree 2 poles (-3.8492, -101.2093) (-3.8589, -100.7619) (-4.2528, -100.2903) (-4.6563, -100.2903) knots 0 0 0 1 2 2 2
  spline S28 degree 2 poles (-4.6563, -100.2903) (-5.0696, -100.2903) (-5.5364, -100.7863) (-5.5607, -101.2093) knots 0 0 0 1 2 2 2
  line L48 (-5.5607, -101.2093) -> (-3.8492, -101.2093)
  line L49 (-0.3241, -104.0537) -> (-1.7341, -104.0537)
  line L50 (-1.7341, -104.0537) -> (-1.7341, -97.7863)
  line L51 (-1.7341, -97.7863) -> (-0.3241, -97.7863)
  line L52 (-0.3241, -97.7863) -> (-0.3241, -104.0537)
  line L53 (5.744, -101.9629) -> (3.0746, -101.9629)
  line L54 (3.0746, -101.9629) -> (3.0746, -100.8446)
  line L55 (3.0746, -100.8446) -> (5.744, -100.8446)
  line L56 (5.744, -100.8446) -> (5.744, -101.9629)
  spline S29 degree 2 poles (11.6565, -104.1801) (10.4458, -104.1801) (9.1427, -103.0132) (9.1427, -101.8851) knots 0 0 0 1 2 2 2
  line L57 (9.1427, -101.8851) -> (9.1427, -98.0537)
  line L58 (9.1427, -98.0537) -> (10.65, -98.0537)
  line L59 (10.65, -98.0537) -> (10.65, -101.7976)
  spline S30 degree 2 poles (10.65, -101.7976) (10.65, -102.4248) (11.1216, -103.0375) (11.6565, -103.0375) knots 0 0 0 1 2 2 2
  spline S31 degree 2 poles (11.6565, -103.0375) (12.1767, -103.0375) (12.6629, -102.4491) (12.6629, -101.7976) knots 0 0 0 1 2 2 2
  line L60 (12.6629, -101.7976) -> (12.6629, -98.0537)
  line L61 (12.6629, -98.0537) -> (14.1702, -98.0537)
  line L62 (14.1702, -98.0537) -> (14.1702, -101.8803)
  spline S32 degree 2 poles (14.1702, -101.8803) (14.1702, -102.9889) (12.9012, -104.1801) (11.6565, -104.1801) knots 0 0 0 1 2 2 2
  spline S33 degree 2 poles (17.9142, -104.1704) (16.5625, -104.1704) (14.9774, -102.5367) (14.9774, -101.0585) knots 0 0 0 1 2 2 2
  spline S34 degree 2 poles (14.9774, -101.0585) (14.9774, -99.6339) (16.5673, -97.937) (17.919, -97.937) knots 0 0 0 1 2 2 2
  spline S35 degree 2 poles (17.919, -97.937) (18.274, -97.937) (18.8477, -98.0196) (19.1103, -98.0877) knots 0 0 0 1 2 2 2
  spline S36 degree 2 poles (19.1103, -98.0877) (19.3145, -98.1509) (19.7959, -98.36) (19.9466, -98.4378) knots 0 0 0 1 2 2 2
  line L63 (19.9466, -98.4378) -> (19.9466, -99.8673)
  line L64 (19.9466, -99.8673) -> (19.7959, -99.8673)
  spline S37 degree 2 poles (19.7959, -99.8673) (19.684, -99.7701) (19.3534, -99.4978) (19.1443, -99.3713) knots 0 0 0 1 2 2 2
  spline S38 degree 2 poles (19.1443, -99.3713) (18.9352, -99.2401) (18.4344, -99.0602) (18.1573, -99.0602) knots 0 0 0 1 2 2 2
  spline S39 degree 2 poles (18.1573, -99.0602) (17.8315, -99.0602) (17.2918, -99.2644) (17.0438, -99.5221) knots 0 0 0 1 2 2 2
  spline S40 degree 2 poles (17.0438, -99.5221) (16.8202, -99.7506) (16.5333, -100.5334) (16.5333, -101.0634) knots 0 0 0 1 2 2 2
  spline S41 degree 2 poles (16.5333, -101.0634) (16.5333, -101.6226) (16.8299, -102.3859) (17.073, -102.6193) knots 0 0 0 1 2 2 2
  spline S42 degree 2 poles (17.073, -102.6193) (17.3064, -102.8478) (17.8801, -103.0472) (18.167, -103.0472) knots 0 0 0 1 2 2 2
  spline S43 degree 2 poles (18.167, -103.0472) (18.4636, -103.0472) (19.0033, -102.8478) (19.1881, -102.7263) knots 0 0 0 1 2 2 2
  spline S44 degree 2 poles (19.1881, -102.7263) (19.3923, -102.6047) (19.6986, -102.347) (19.8104, -102.2449) knots 0 0 0 1 2 2 2
  line L65 (19.8104, -102.2449) -> (19.9466, -102.2449)
  line L66 (19.9466, -102.2449) -> (19.9466, -103.655)
  spline S45 degree 2 poles (19.9466, -103.655) (19.7813, -103.7328) (19.3485, -103.9273) (19.1151, -103.9953) knots 0 0 0 1 2 2 2
  spline S46 degree 2 poles (19.1151, -103.9953) (18.8331, -104.0829) (18.342, -104.1704) (17.9142, -104.1704) knots 0 0 0 1 2 2 2
  line L67 (24.9887, -99.5269) -> (23.3647, -104.0537)
  line L68 (23.3647, -104.0537) -> (21.8234, -104.0537)
  line L69 (21.8234, -104.0537) -> (20.214, -99.5269)
  line L70 (20.214, -99.5269) -> (21.697, -99.5269)
  line L71 (21.697, -99.5269) -> (22.6208, -102.5172)
  line L72 (22.6208, -102.5172) -> (23.5349, -99.5269)
  line L73 (23.5349, -99.5269) -> (24.9887, -99.5269)
  constraints: 2 other
emboss "Emboss1" sketch "Sketch20" operation add depth 1 direction (0, 0, -1)
equation "\"d17\" = DiaGauri"
equation "\"d26\" = DiaGauri"
equation "\"d35\" = DiaGauri"
equation "\"d44\" = DiaGauri"
equation "\"d53\" = DiaGauri"
equation "\"d62\" = DiaGauri"
equation "\"d71\" = DiaGauri"
equation "\"d80\" = DiaGauri"
equation "\"d89\" = DiaGauri"
equation "\"d98\" = DiaGauri"
equation "\"d107\" = DiaGauri"
equation "\"d116\" = DiaGauri"
equation "\"d125\" = DiaGauri"
equation "\"d192\" = d191"
equation "\"DiaGauri\" = 10"
body "Solid1"
